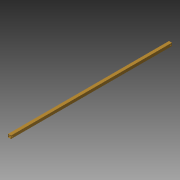
# Autodesk Inventor part: Arm
Saved by Autodesk Inventor 2015 (Build 190159000, 159)
## iProperties
Created: 2015-02-07
Part Number: Arm
Material: Brass, Soft Yellow
Document SubType Name: Modeling
Designer: pltwe4
Density: 8.47 g/cm^3
Appearance: Brass - Satin
Author: pltwe4
Autodesk Inventor part; units mm, degrees
ref_plane "YZ Plane" through (0, 0, 0) normal (1, 0, 0) x (0, 1, 0)
ref_plane "XZ Plane" through (0, 0, 0) normal (0, 1, 0) x (-1, 0, 0)
ref_plane "XY Plane" through (0, 0, 0) normal (0, 0, 1) x (1, 0, 0)
sketch "Sketch1" plane through (0, 0, 0) normal (0, 0, 1) x (1, 0, 0)
  line L0 (-12.7, 12.7) -> (12.7, 12.7)
  line L1 (12.7, 12.7) -> (12.7, -12.7)
  line L2 (12.7, -12.7) -> (-12.7, -12.7)
  line L3 (-12.7, -12.7) -> (-12.7, 12.7)
  line L4 (-17.78, 0) -> (17.78, 0) projected
  line L5 (0, 17.78) -> (0, -17.78) projected
  line L6 (11.43, 11.43) -> (-11.43, 11.43)
  line L7 (-11.43, 11.43) -> (-11.43, -11.43)
  line L8 (-11.43, -11.43) -> (11.43, -11.43)
  line L9 (11.43, -11.43) -> (11.43, 11.43)
  point P0 (0, 0)
  dimension "d0" = 25.4
  dimension "d1" = 1.27
  constraints: 16 end point, 4 parallel, 3 perpendicular, 1 horizontal, 5 other
  measures "d0" distance of L0.start L0.end
  measures "d1" distance between parallel lines of L0 L6
extrude "Extrusion1" add sketch "Sketch1" along normal mid plane 1397 contours L0 L5 L6 L7 L4 L3 | L0 L1 L4 L9 L6 L5 | L4 L7 L8 L5 L2 L3 | L1 L2 L5 L8 L9 L4
sketch "Sketch2" plane through (12.7, 12.7, 698.5) normal (1, 0, 0) x (0, 0, -1)
  line L0 (0, 0) -> (1397, 0) projected
  line L1 (0, -25.4) -> (0, 0) projected
  line L2 (0, -25.4) -> (1397, -25.4) projected
  line L3 (1397, 0) -> (1397, -25.4) projected
  circle A0 centre (9.525, -12.7) radius 4.7625
  circle A1 centre (1387.475, -12.7) radius 4.7625
  line L4 (698.5, -30.48) -> (698.5, 5.08) projected
  point P0 (698.5, -12.7)
  dimension "d4" = 9.525
  dimension "d5" = 9.525
  dimension "d6" = 12.7
  constraints: 2 centre point, 1 other
  measures "d4" diameter of A0
  measures "d5" distance from line of L1 A0.centre
  measures "d6" distance from line of L0 A0.centre
extrude "Extrusion2" cut sketch "Sketch2" against normal up to surface (25.4 mm away) contours A0 | A1
equation "\"d2\" = ArmLength"
equation "\"d7\" = ArmLength"
equation "\"ArmLength\" = 1397"
body "Solid1"
